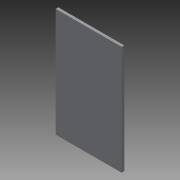
# Autodesk Inventor part: blacha pion rbc
Saved by Autodesk Inventor 2015 (Build 190159000, 159)
## iProperties
Created: 2015-05-04
Part Number: blacha pion rbc
Material: Ogólny
Document SubType Name: Modeling
Designer: Kuba
Density: 1 g/cm^3
Appearance: Domyślna
Author: Kuba
Autodesk Inventor part; units mm, degrees
ref_plane "YZ Plane" through (0, 0, 0) normal (1, 0, 0) x (0, 1, 0)
ref_plane "XZ Plane" through (0, 0, 0) normal (0, 1, 0) x (-1, 0, 0)
ref_plane "XY Plane" through (0, 0, 0) normal (0, 0, 1) x (1, 0, 0)
sketch "Szkic1" plane through (0, 0, 0) normal (0, 1, 0) x (-1, 0, 0)
  line L0 (-25, -41.4) -> (25, -41.4)
  line L1 (25, -41.4) -> (25, 41.4)
  line L2 (25, 41.4) -> (-25, 41.4)
  line L3 (-25, 41.4) -> (-25, -41.4)
  line L4 (-25, -41.4) -> (25, 41.4) construction
  line L5 (25, -41.4) -> (-25, 41.4) construction
  point P0 (0, 0)
  dimension "d0" = 50
  dimension "d1" = 82.8
  constraints: 12 end point, 2 midpoint, 2 parallel, 1 horizontal, 1 perpendicular
  measures "d0" distance of L2.end L1.end
  measures "d1" distance of L1.end L0.end
extrude "Wyciągnięcie proste1" add sketch "Szkic1" along normal blind 2
sketch "Szkic3" plane through (0, 0, 0) normal (0, -1, 0) x (1, 0, 0)
  circle A0 centre (-19.4, 16.1) radius 1.75 projected
  circle A1 centre (16.6, -37.9) radius 1.75 projected
  line L0 (20.1, -41.4) -> (-25, -41.4) projected
  line L1 (20.1, 41.4) -> (20.1, -41.4) projected
  line L2 (-25, 41.4) -> (20.1, 41.4) projected
  line L3 (-25, -41.4) -> (-25, 41.4) projected
  point P0 (0, 0)
hole "Otwór1" at (16.6, 0, -37.9) at (-19.4, 0, 16.1) direction (0, 1, 0) diameter 3.5 end through all
